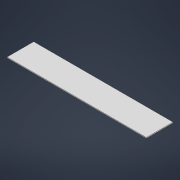
# Autodesk Inventor part: goalPanelTop
Saved by Autodesk Inventor 2021 (Build 250183000, 183)
## iProperties
Created: 2021-11-24
Part Number: goalPanelTop
Material: Generic
Document SubType Name: Modeling
Designer: jo_ki
Density: 1 g/cm^3
Appearance: Default
Author: jo_ki
Autodesk Inventor part; units mm, degrees
ref_plane "YZ Plane" through (0, 0, 0) normal (1, 0, 0) x (0, 1, 0)
ref_plane "XZ Plane" through (0, 0, 0) normal (0, 1, 0) x (-1, 0, 0)
ref_plane "XY Plane" through (0, 0, 0) normal (0, 0, 1) x (1, 0, 0)
sketch "Sketch1" plane through (0, 0, 0) normal (0, 1, 0) x (-1, 0, 0)
  line L0 (-340, 65) -> (340, 65)
  line L1 (340, 65) -> (340, -65)
  line L2 (340, -65) -> (-340, -65)
  line L3 (-340, -65) -> (-340, 65)
  line L4 (-340, 65) -> (340, -65) construction
  line L5 (340, 65) -> (-340, -65) construction
  point P0 (0, 0)
  dimension "d1" = 680
  dimension "d2" = 130
  constraints: 12 end point, 2 midpoint, 2 parallel, 1 horizontal, 1 perpendicular
  measures "d1" distance of L0.start L0.end
  measures "d2" distance of L0.end L1.end
derived "Mastersketch.ipt"
extrude "Extrusion1" add sketch "Sketch1" along normal blind 4
equation "\"d1\" = feet_widthCenter - profile_width"
equation "\"d2\" = -0.5 * glass_length + 0.5 * feet_lengthCenter - 0.5 * profile_width"
equation "\"d3\" = goalPanel_thickness"
equation "\"feet_widthCenter\" = 720"
equation "\"profile_width\" = 40"
equation "\"glass_length\" = 1200"
equation "\"feet_lengthCenter\" = 1500"
equation "\"goalPanel_thickness\" = 4"
body "Solid1"
